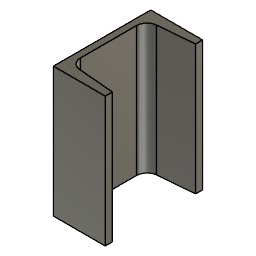
C-75×40×5×7 (Autodesk Fusion 360 design; units mm, degrees)
Autodesk Fusion 360 part; units mm, degrees
note: some values were not read from the file. Set by a fixed rule: which sketch regions a step uses.
sketch "スケッチ1" plane through (0, 0, 0) normal (0, 0, 1) x (1, 0, 0)
  line L0 (0, 75) -> (0, 0)
  line L1 (0, 0) -> (40, 0)
  line L2 (40, 5.4689) -> (40, 0)
  line L3 (5, 59.1383) -> (5, 15.8617)
  line L4 (12.3028, 7.8921) -> (40, 5.4689)
  arc A0 (5, 15.8617) -> (12.3028, 7.8921) centre (13, 15.8617) ccw
  line L5 (40, 69.5311) -> (12.3028, 67.1079)
  arc A1 (12.3028, 67.1079) -> (5, 59.1383) centre (13, 59.1383) ccw
  line L6 (0, 75) -> (40, 75)
  line L7 (40, 75) -> (40, 69.5311)
extrude "押し出し1" add sketch "スケッチ1" along normal blind 100
